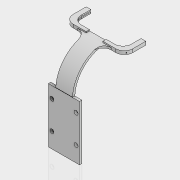
# Autodesk Inventor part: ЛЦМК000002.00.00.00.00.14-01 Фиксатор OLED
Saved by Autodesk Inventor 2021.2 (Build 252289000, 289)
## iProperties
Created: 2025-11-04
Part Number: ЛЦМК000002.00.00.00.00.14-01 Фиксатор OLED
Material: Типовые
Document SubType Name: Modeling
Designer: Захаров
Density: 1 g/cm^3
Appearance: По умолчанию
Author: Захаров
Autodesk Inventor part; units mm, degrees
ref_plane "YZ Plane" through (0, 0, 0) normal (1, 0, 0) x (0, 1, 0)
ref_plane "XZ Plane" through (0, 0, 0) normal (0, 1, 0) x (-1, 0, 0)
ref_plane "XY Plane" through (0, 0, 0) normal (0, 0, 1) x (1, 0, 0)
sketch "Эскиз1" plane through (0, 0, 0) normal (0, 0, 1) x (1, 0, 0)
  line L0 (7.65, 12.3) -> (7.65, 19.5) projected
  line L1 (7.65, 19.5) -> (11.5, 19.5) projected
  line L2 (11.5, 19.5) -> (11.5, -21.5) projected
  line L3 (11.5, -21.5) -> (9, -21.5) projected
  line L4 (9, -21.5) -> (9, -13.3) projected
  line L5 (9, -13.3) -> (-9, -13.3) projected
  line L6 (-9, -13.3) -> (-9, -21.5) projected
  line L7 (-9, -21.5) -> (-11.7, -21.5) projected
  line L8 (-11.7, -21.5) -> (-11.7, 19.5) projected
  line L9 (-11.7, 19.5) -> (-7.85, 19.5) projected
  line L10 (-7.85, 19.5) -> (-7.85, 12.3) projected
  line L11 (-7.85, 12.3) -> (7.65, 12.3) projected
  circle A0 centre (9, 11.0154) radius 1.5 projected
  circle A1 centre (-9, -9.9846) radius 1.5 projected
  circle A2 centre (9, -9.9846) radius 1.5 projected
  circle A3 centre (-9, 11.0154) radius 1.5 projected
  line L12 (-9, -21.5) -> (9, -21.5)
  line L13 (7.65, 19.5) -> (-7.85, 19.5)
  point P0 (0, 0)
  constraints: 4 end point, 1 horizontal, 1 perpendicular
extrude "Выдавливание1" add sketch "Эскиз1" along normal blind 1.8
sketch "Эскиз2" plane through (-11.7, 19.5, 0) normal (0, 1, 0) x (1, 0, 0)
  line L0 (17.95, -1.7) -> (5.45, -1.7)
  line L1 (5.45, -1.7) -> (5.45, 0)
  line L2 (5.45, 0) -> (17.95, 0)
  line L3 (17.95, 0) -> (17.95, -1.7)
  point P0 (11.7, 0)
  point P1 (11.7, 0)
  dimension "d2" = 12.5
  dimension "d3" = 1.7
  constraints: 8 end point, 2 parallel, 1 coincident, 1 horizontal, 1 midpoint, 1 perpendicular
  measures "d2" distance of L1.end L2.end
  measures "d3" distance of L0.end L1.end
sketch "Эскиз3" plane through (0, 0, 0) normal (1, 0, 0) x (0, 1, 0)
  line L0 (19.5, 0) -> (-21.5, 0) projected
  arc A0 (41.9054, -23.4745) -> (19.5, 0) centre (18.4054, -23.4745) ccw
  line L1 (45.943, -23.4745) -> (37.8678, -23.4745) construction
  point P0 (0, 0)
  dimension "d4" = 23.5
  constraints: 2 end point, 2 point on circle, 1 centre point, 1 horizontal, 1 line through centre, 1 midpoint
  measures "d4" radius of A0
sweep "Сдвиг1" add profiles "Эскиз2" path "Эскиз3" path curves A0 L0
sketch "Эскиз4" plane through (6.25, 41.9054, -23.4745) normal (1, 0, 0) x (0, 0, -1)
  line L0 (0, 0) -> (-2.5, 0)
  line L1 (-2.5, 0) -> (-2.5, 2.5206)
  line L2 (-2.5, 2.5206) -> (0, 2.5206)
  line L3 (0, 2.5206) -> (0, 0)
  point P0 (-23.4745, -41.9054)
  dimension "d7" = 2.5
  constraints: 8 end point, 2 parallel, 1 horizontal, 1 perpendicular
  measures "d7" distance of L1.end L2.end
extrude "Выдавливание2" add sketch "Эскиз4" along normal blind 16
sketch "Эскиз5" plane through (-6.25, 41.9054, -23.4745) normal (0, 0, -1) x (-1, 0, 0)
  line L0 (-12.5, 2.5206) -> (-28.5, 2.5206) projected
  line L1 (-12.5, 0) -> (-28.5, 0) projected
  line L2 (-28.5, 2.5206) -> (-25, 2.5206)
  line L3 (-25, 2.5206) -> (-25, 0)
  line L4 (-25, 0) -> (-28.5, 0)
  line L5 (-28.5, 0) -> (-28.5, 2.5206)
  line L6 (-25, 0.9103) -> (-28.5, 0.9103)
  line L7 (-28.5, 0.9103) -> (-28.5, 1.6103)
  line L8 (-28.5, 1.6103) -> (-25, 1.6103)
  line L9 (-25, 1.6103) -> (-25, 0.9103)
  line L10 (-28.5, 0) -> (-28.5, 2.5206) projected
  line L11 (-28.5, 1.6103) -> (-27.5, 1.6103)
  line L12 (-27.5, 1.6103) -> (-27.5, 0.9103)
  line L13 (-28.5, 1.6413) -> (-28.5, 1.6103)
  point P0 (-6.25, -41.9054)
  point P1 (-28.5, 1.2603)
  point P2 (-27.5, 1.6103)
  dimension "d10" = 3.5
  dimension "d11" = 0.7
  dimension "d13" = 1
  constraints: 22 end point, 5 parallel, 4 point on line, 3 horizontal, 3 perpendicular, 2 midpoint
  measures "d10" distance of L3.end L4.end
  measures "d11" distance of L6.end L7.end
  measures "d13" distance from line of L13.start L12
extrude "Выдавливание3" add sketch "Эскиз5" along normal blind 13.5 contours L3 L8 L5 L0 | L3 L1 L5 L6 | L12 L6 L5 L8
mirror "Зеркальное отражение1" about plane through (0, 0, 0) normal (1, 0, 0) of "Выдавливание3", "Выдавливание2"
fillet "Сопряжение1" radius 6.25 6 edges at (6.25, 42.6932, -20.9745) (-6.25, 42.6932, -20.9745) (18.75, 43.9708, -23.4745) (-18.75, 43.9708, -23.4745) (-18.75, 42.3605, -23.4745) (18.75, 42.3605, -23.4745)
fillet "Сопряжение2" radius 6.25 2 edges at (22.25, 43.1657, -20.9745) (-22.25, 43.1657, -20.9745)
